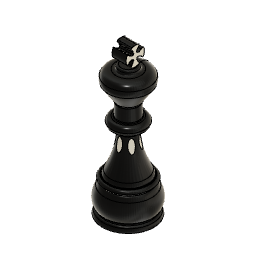
King (Autodesk Fusion 360 design; units mm, degrees)
Autodesk Fusion 360 part; units mm, degrees
(part 1 of 2)
sketch "King" plane through (0, 0, 0) normal (1, 0, 0) x (0, 1, 0)
  spline S0 degree 3 poles (88.295222, 49.849064) (89.98216, 50.061446) (91.649324, 49.850976) (93.310746, 49.908379) knots 0 0 0 0 1 1 1 1
  spline S1 degree 3 poles (93.310746, 49.908379) (93.855415, 49.926874) (93.710002, 49.535914) (93.695969, 49.290366) knots 0 0 0 0 1 1 1 1
  spline S2 degree 3 poles (93.695969, 49.290366) (93.638571, 48.352187) (93.519308, 47.4172) (93.457443, 46.479021) knots 0 0 0 0 1 1 1 1
  spline S3 degree 3 poles (93.457443, 46.479021) (93.421085, 45.919049) (93.415353, 45.480889) (94.299953, 45.59569) knots 0 0 0 0 1 1 1 1
  spline S4 degree 3 poles (94.299953, 45.59569) (94.931994, 45.677326) (95.640576, 45.650539) (96.29175, 45.57847) knots 0 0 0 0 1 1 1 1
  spline S5 degree 3 poles (96.29175, 45.57847) (97.320498, 45.464306) (97.41042, 45.937544) (97.282865, 46.743702) knots 0 0 0 0 1 1 1 1
  spline S6 degree 3 poles (97.282865, 46.743702) (97.158493, 47.528177) (97.128519, 48.328592) (96.995865, 49.11115) knots 0 0 0 0 1 1 1 1
  spline S7 degree 3 poles (96.995865, 49.11115) (96.893817, 49.711943) (97.141277, 49.926237) (97.686579, 49.925599) knots 0 0 0 0 1 1 1 1
  spline S8 degree 3 poles (97.686579, 49.925599) (99.190472, 49.923687) (100.69564, 49.921133) (102.198258, 49.912204) knots 0 0 0 0 1 1 1 1
  spline S9 degree 3 poles (102.198258, 49.912204) (102.707844, 49.909654) (102.999312, 49.79804) (102.885148, 49.134745) knots 0 0 0 0 1 1 1 1
  spline S10 degree 3 poles (102.885148, 49.134745) (102.473143, 46.743697) (101.897225, 44.366044) (100.371007, 42.473103) knots 0 0 0 0 1 1 1 1
  spline S11 degree 3 poles (100.371007, 42.473103) (99.617786, 41.540028) (98.842239, 40.438574) (97.084512, 40.530413) knots 0 0 0 0 1 1 1 1
  spline S12 degree 3 poles (97.084512, 40.530413) (92.929989, 40.747257) (88.756976, 40.584629) (84.591622, 40.565486) knots 0 0 0 0 1 1 1 1
  spline S13 degree 3 poles (84.591622, 40.565486) (83.961488, 40.562937) (83.402153, 40.683475) (82.942949, 41.155437) knots 0 0 0 0 1 1 1 1
  spline S14 degree 3 poles (82.942949, 41.155437) (80.750249, 43.416377) (79.704928, 46.184994) (79.359887, 49.260383) knots 0 0 0 0 1 1 1 1
  spline S15 degree 3 poles (79.359887, 49.260383) (79.326088, 49.555674) (79.183858, 49.961305) (79.775717, 49.951102) knots 0 0 0 0 1 1 1 1
  spline S16 degree 3 poles (79.775717, 49.951102) (81.317243, 49.924315) (82.860034, 49.928777) (84.402193, 49.924952) knots 0 0 0 0 1 1 1 1
  spline S17 degree 3 poles (84.402193, 49.924952) (84.984485, 49.92304) (85.252995, 49.714483) (85.154772, 49.063946) knots 0 0 0 0 1 1 1 1
  spline S18 degree 3 poles (85.154772, 49.063946) (85.015101, 48.136608) (84.967259, 47.195242) (84.870321, 46.26153) knots 0 0 0 0 1 1 1 1
  spline S19 degree 3 poles (84.870321, 46.26153) (84.830138, 45.887153) (84.860112, 45.517875) (85.334625, 45.564432) knots 0 0 0 0 1 1 1 1
  spline S20 degree 3 poles (85.334625, 45.564432) (86.334032, 45.663925) (87.34173, 45.403711) (88.341136, 45.668392) knots 0 0 0 0 1 1 1 1
  spline S21 degree 3 poles (88.341136, 45.668392) (88.594338, 45.735999) (88.788857, 45.702833) (88.752509, 46.051061) knots 0 0 0 0 1 1 1 1
  spline S22 degree 3 poles (88.752509, 46.051061) (88.619845, 47.303674) (88.682985, 48.578597) (88.295222, 49.849064) knots 0 0 0 0 1 1 1 1
  spline S23 degree 3 poles (32.804917, 55.77343) (30.85904, 55.684778) (28.973753, 57.437406) (28.855127, 59.445149) knots 0 0 0 0 1 1 1 1
  spline S24 degree 3 poles (28.855127, 59.445149) (28.719281, 61.741804) (30.431727, 63.767404) (32.57914, 63.848401) knots 0 0 0 0 1 1 1 1
  spline S25 degree 3 poles (32.57914, 63.848401) (34.856025, 63.933866) (36.967084, 62.39362) (36.930731, 59.527421) knots 0 0 0 0 1 1 1 1
  spline S26 degree 3 poles (36.930731, 59.527421) (36.909049, 57.853236) (35.523786, 55.816157) (32.804917, 55.77343) knots 0 0 0 0 1 1 1 1
  spline S27 degree 3 poles (-3.40457, 66.888069) (-2.853527, 66.263682) (-2.253372, 65.822973) (-1.529489, 65.53533) knots 0 0 0 0 1 1 1 1
  spline S28 degree 3 poles (-1.529489, 65.53533) (-1.252053, 65.424996) (-1.000768, 65.382901) (-0.766702, 65.520659) knots 0 0 0 0 1 1 1 1
  spline S29 degree 3 poles (-0.766702, 65.520659) (-0.442708, 65.713271) (-0.529445, 66.069153) (-0.5945, 66.342763) knots 0 0 0 0 1 1 1 1
  spline S30 degree 3 poles (-0.5945, 66.342763) (-0.736088, 66.937813) (-1.02564, 67.460157) (-1.505255, 67.870888) knots 0 0 0 0 1 1 1 1
  spline S31 degree 3 poles (-1.505255, 67.870888) (-1.91535, 68.222308) (-1.795447, 68.486346) (-1.331778, 68.68215) knots 0 0 0 0 1 1 1 1
  spline S32 degree 3 poles (-1.331778, 68.68215) (-0.632768, 68.976804) (0.116627, 69.05589) (0.833495, 68.955759) knots 0 0 0 0 1 1 1 1
  spline S33 degree 3 poles (0.833495, 68.955759) (2.154343, 68.770164) (2.208554, 68.532908) (1.445766, 67.461432) knots 0 0 0 0 1 1 1 1
  spline S34 degree 3 poles (1.445766, 67.461432) (1.069476, 66.932709) (0.436793, 66.287272) (1.044602, 65.686484) knots 0 0 0 0 1 1 1 1
  spline S35 degree 3 poles (1.044602, 65.686484) (1.70343, 65.034668) (2.367362, 65.740695) (2.894811, 66.132293) knots 0 0 0 0 1 1 1 1
  spline S36 degree 3 poles (2.894811, 66.132293) (3.795999, 66.80133) (4.067054, 66.782192) (4.250099, 65.699238) knots 0 0 0 0 1 1 1 1
  spline S37 degree 3 poles (4.250099, 65.699238) (4.392962, 64.851623) (4.480339, 63.975946) (4.074071, 63.130886) knots 0 0 0 0 1 1 1 1
  spline S38 degree 3 poles (4.074071, 63.130886) (3.839369, 62.642982) (3.686298, 62.435705) (3.265363, 62.970165) knots 0 0 0 0 1 1 1 1
  spline S39 degree 3 poles (3.265363, 62.970165) (2.882695, 63.454244) (2.348229, 63.767394) (1.75892, 63.931944) knots 0 0 0 0 1 1 1 1
  spline S40 degree 3 poles (1.75892, 63.931944) (1.06246, 64.12583) (0.724436, 63.78079) (0.87049, 63.076037) knots 0 0 0 0 1 1 1 1
  spline S41 degree 3 poles (0.87049, 63.076037) (1.013353, 62.387868) (1.479574, 61.888486) (1.897321, 61.366142) knots 0 0 0 0 1 1 1 1
  spline S42 degree 3 poles (1.897321, 61.366142) (2.223867, 60.957961) (2.184322, 60.770454) (1.632641, 60.628228) knots 0 0 0 0 1 1 1 1
  spline S43 degree 3 poles (1.632641, 60.628228) (0.702753, 60.387785) (-0.209914, 60.262143) (-1.138527, 60.583584) knots 0 0 0 0 1 1 1 1
  spline S44 degree 3 poles (-1.138527, 60.583584) (-1.749523, 60.795328) (-2.119436, 61.023018) (-1.449127, 61.670367) knots 0 0 0 0 1 1 1 1
  spline S45 degree 3 poles (-1.449127, 61.670367) (-1.077937, 62.028799) (-0.866832, 62.561352) (-0.617457, 63.03331) knots 0 0 0 0 1 1 1 1
  spline S46 degree 3 poles (-0.617457, 63.03331) (-0.483523, 63.287149) (-0.537734, 63.575424) (-0.729706, 63.787806) knots 0 0 0 0 1 1 1 1
  spline S47 degree 3 poles (-0.729706, 63.787806) (-0.92997, 64.009754) (-1.17743, 64.010392) (-1.462518, 63.889212) knots 0 0 0 0 1 1 1 1
  spline S48 degree 3 poles (-1.462518, 63.889212) (-2.044175, 63.641752) (-2.652621, 63.454244) (-3.078022, 62.939554) knots 0 0 0 0 1 1 1 1
  spline S49 degree 3 poles (-3.078022, 62.939554) (-3.416047, 62.530736) (-3.63417, 62.686352) (-3.768741, 63.111753) knots 0 0 0 0 1 1 1 1
  spline S50 degree 3 poles (-3.768741, 63.111753) (-4.167358, 64.373933) (-4.231775, 65.608679) (-3.40457, 66.888069) knots 0 0 0 0 1 1 1 1
  spline S51 degree 3 poles (134.32848, 40.360768) (132.205294, 41.878052) (130.602545, 43.799055) (129.497266, 46.158212) knots 0 0 0 0 1 1 1 1
  spline S52 degree 3 poles (129.497266, 46.158212) (129.186024, 46.822145) (128.865867, 47.537738) (128.279741, 47.989289) knots 0 0 0 0 1 1 1 1
  spline S53 degree 3 poles (128.279741, 47.989289) (127.659826, 48.466351) (127.314133, 48.86879) (127.629832, 49.724696) knots 0 0 0 0 1 1 1 1
  spline S54 degree 3 poles (127.629832, 49.724696) (127.886868, 50.42052) (127.423187, 51.113151) (126.876611, 51.455637) knots 0 0 0 0 1 1 1 1
  spline S55 degree 3 poles (126.876611, 51.455637) (126.403373, 51.752204) (126.004759, 51.185857) (125.676311, 50.811475) knots 0 0 0 0 1 1 1 1
  spline S56 degree 3 poles (125.676311, 50.811475) (125.337644, 50.426894) (124.966454, 50.359925) (124.427527, 50.451764) knots 0 0 0 0 1 1 1 1
  spline S57 degree 3 poles (124.427527, 50.451764) (121.666568, 50.923084) (119.036346, 50.471534) (116.559838, 49.154515) knots 0 0 0 0 1 1 1 1
  spline S58 degree 3 poles (116.559838, 49.154515) (114.237666, 47.919769) (112.702524, 46.003866) (111.62467, 43.63833) knots 0 0 0 0 1 1 1 1
  spline S59 degree 3 poles (111.62467, 43.63833) (110.243232, 40.608861) (109.600349, 37.40783) (109.385413, 34.123885) knots 0 0 0 0 1 1 1 1
  spline S60 degree 3 poles (109.385413, 34.123885) (109.150069, 30.51914) (109.299948, 26.913744) (110.003421, 23.361931) knots 0 0 0 0 1 1 1 1
  spline S61 degree 3 poles (110.003421, 23.361931) (110.380985, 21.456231) (110.852306, 19.571591) (111.717783, 17.794721) knots 0 0 0 0 1 1 1 1
  spline S62 degree 3 poles (111.717783, 17.794721) (112.014992, 17.181813) (112.370874, 16.874405) (112.900868, 16.769808) knots 0 0 0 0 1 1 1 1
  line L0 (112.900868, 16.769808) -> (128.298854, 16.769808)
  spline S63 degree 3 poles (128.298854, 16.769808) (128.712144, 16.855905) (128.881789, 17.128239) (128.935995, 17.633368) knots 0 0 0 0 1 1 1 1
  spline S64 degree 3 poles (128.935995, 17.633368) (129.147097, 19.555651) (129.375424, 21.475374) (129.624792, 23.391915) knots 0 0 0 0 1 1 1 1
  spline S65 degree 3 poles (129.624792, 23.391915) (129.697508, 23.948057) (129.53232, 24.320522) (129.118388, 24.708296) knots 0 0 0 0 1 1 1 1
  spline S66 degree 3 poles (129.118388, 24.708296) (127.229272, 26.471123) (125.479845, 28.356414) (124.242545, 30.660086) knots 0 0 0 0 1 1 1 1
  spline S67 degree 3 poles (124.242545, 30.660086) (122.998238, 32.979698) (122.026245, 35.380318) (121.938873, 38.058372) knots 0 0 0 0 1 1 1 1
  spline S68 degree 3 poles (121.938873, 38.058372) (121.92484, 38.469102) (122.016046, 39.016321) (122.367462, 39.04757) knots 0 0 0 0 1 1 1 1
  spline S69 degree 3 poles (122.367462, 39.04757) (122.838149, 39.08966) (122.728453, 38.509285) (122.7935, 38.170618) knots 0 0 0 0 1 1 1 1
  spline S70 degree 3 poles (122.7935, 38.170618) (123.213154, 35.969627) (124.448547, 35.266796) (126.661655, 35.799982) knots 0 0 0 0 1 1 1 1
  spline S71 degree 3 poles (126.661655, 35.799982) (128.582653, 36.262379) (130.517061, 36.572979) (132.13575, 34.857974) knots 0 0 0 0 1 1 1 1
  spline S72 degree 3 poles (132.13575, 34.857974) (132.348779, 34.632196) (133.05161, 34.012271) (133.616677, 34.937054) knots 0 0 0 0 1 1 1 1
  spline S73 degree 3 poles (133.616677, 34.937054) (134.08353, 35.698567) (134.68624, 36.385457) (135.069556, 37.214576) knots 0 0 0 0 1 1 1 1
  spline S74 degree 3 poles (135.069556, 37.214576) (135.723941, 38.62919) (135.575337, 39.469151) (134.32848, 40.360768) knots 0 0 0 0 1 1 1 1
  line L1 (102.334737, 3.260296) -> (79.669845, 3.260296)
  spline S75 degree 3 poles (79.669845, 3.260296) (78.967647, 3.011561) (78.601556, 2.40056) (78.233558, 1.257016) knots 0 0 0 0 1 1 1 1
  spline S76 degree 3 poles (78.233558, 1.257016) (77.972065, 0.443846) (78.199117, 0.343706) (78.894298, 0.345623) knots 0 0 0 0 1 1 1 1
  spline S77 degree 3 poles (78.894298, 0.345623) (82.659131, 0.359656) (86.423963, 0.359014) (90.188153, 0.356464) knots 0 0 0 0 1 1 1 1
  spline S78 degree 3 poles (90.188153, 0.356464) (94.570994, 0.353272) (98.951926, 0.354547) (103.332859, 0.325216) knots 0 0 0 0 1 1 1 1
  spline S79 degree 3 poles (103.332859, 0.325216) (104.040799, 0.320116) (104.111588, 0.614133) (103.980208, 1.194518) knots 0 0 0 0 1 1 1 1
  spline S80 degree 3 poles (103.980208, 1.194518) (103.707884, 2.394185) (103.22508, 3.025594) (102.334737, 3.260296) knots 0 0 0 0 1 1 1 1
  spline S81 degree 3 poles (38.99141, 16.190708) (39.060291, 16.192625) (39.129173, 16.195807) (39.19805, 16.199641) knots 0 0 0 0 1 1 1 1
  spline S82 degree 3 poles (39.19805, 16.199641) (39.19805, 16.196449) (39.19805, 16.193267) (39.19805, 16.190708) knots 0 0 0 0 1 1 1 1
  line L2 (39.19805, 16.190708) -> (41.8002, 16.190708)
  spline S83 degree 3 poles (41.8002, 16.190708) (42.145883, 17.004519) (41.415619, 17.417799) (41.11841, 17.961826) knots 0 0 0 0 1 1 1 1
  spline S84 degree 3 poles (41.11841, 17.961826) (38.833234, 22.135481) (37.535348, 26.59677) (36.994504, 31.315084) knots 0 0 0 0 1 1 1 1
  spline S85 degree 3 poles (36.994504, 31.315084) (36.870774, 32.396131) (36.972179, 33.513526) (36.581219, 34.669819) knots 0 0 0 0 1 1 1 1
  line L3 (36.581219, 34.669819) -> (28.943769, 34.669819)
  spline S86 degree 3 poles (28.943769, 34.669819) (28.773483, 34.470833) (28.714167, 34.199773) (28.696309, 33.859832) knots 0 0 0 0 1 1 1 1
  spline S87 degree 3 poles (28.696309, 33.859832) (28.545155, 30.988534) (28.07128, 28.161243) (27.40799, 25.367119) knots 0 0 0 0 1 1 1 1
  spline S88 degree 3 poles (27.40799, 25.367119) (26.631806, 22.092107) (24.830709, 19.246316) (23.532823, 16.190698) knots 0 0 0 0 1 1 1 1
  line L4 (23.532823, 16.190698) -> (38.99141, 16.190708)
  spline S89 degree 3 poles (42.254305, 15.822067) (42.187973, 15.826534) (42.091667, 15.824617) (41.998554, 15.828442) knots 0 0 0 0 1 1 1 1
  line L5 (41.998554, 15.828442) -> (23.18587, 15.828442)
  spline S90 degree 3 poles (23.18587, 15.828442) (23.118901, 15.813776) (23.04747, 15.808667) (22.976676, 15.808034) knots 0 0 0 0 1 1 1 1
  spline S91 degree 3 poles (22.976676, 15.808034) (22.224092, 15.801017) (21.936454, 15.235941) (21.968978, 14.682348) knots 0 0 0 0 1 1 1 1
  spline S92 degree 3 poles (21.968978, 14.682348) (22.010435, 13.994183) (22.542346, 13.769038) (23.270693, 13.771598) knots 0 0 0 0 1 1 1 1
  spline S93 degree 3 poles (23.270693, 13.771598) (29.545199, 13.792647) (35.820348, 13.775422) (42.09485, 13.759481) knots 0 0 0 0 1 1 1 1
  spline S94 degree 3 poles (42.09485, 13.759481) (42.725616, 13.758207) (43.304726, 13.900427) (43.386356, 14.585409) knots 0 0 0 0 1 1 1 1
  spline S95 degree 3 poles (43.386356, 14.585409) (43.475023, 15.334806) (43.04261, 15.77551) (42.254305, 15.822067) knots 0 0 0 0 1 1 1 1
  line L6 (83.250357, 37.423138) -> (98.576921, 37.423138)
  spline S96 degree 3 poles (98.576921, 37.423138) (98.641336, 37.430155) (98.704476, 37.435897) (98.768258, 37.446096) knots 0 0 0 0 1 1 1 1
  spline S97 degree 3 poles (98.768258, 37.446096) (99.605669, 37.575567) (100.289367, 38.34218) (100.172654, 39.018228) knots 0 0 0 0 1 1 1 1
  spline S98 degree 3 poles (100.172654, 39.018228) (100.026599, 39.866481) (99.518288, 40.270194) (98.631128, 40.26637) knots 0 0 0 0 1 1 1 1
  spline S99 degree 3 poles (98.631128, 40.26637) (93.665353, 40.240863) (88.699568, 40.230012) (83.734436, 40.230012) knots 0 0 0 0 1 1 1 1
  spline S100 degree 3 poles (83.734436, 40.230012) (83.081345, 40.230012) (82.538593, 40.070566) (82.266258, 39.448091) knots 0 0 0 0 1 1 1 1
  spline S101 degree 3 poles (82.266258, 39.448091) (81.891876, 38.592199) (82.384247, 37.714606) (83.250357, 37.423138) knots 0 0 0 0 1 1 1 1
  spline S102 degree 3 poles (99.326309, 26.046369) (98.959585, 29.268449) (98.668118, 32.494987) (98.36326, 35.721534) knots 0 0 0 0 1 1 1 1
  spline S103 degree 3 poles (98.36326, 35.721534) (98.275888, 36.648867) (98.229963, 36.960109) (97.7816, 37.060882) knots 0 0 0 0 1 1 1 1
  line L7 (97.7816, 37.060882) -> (84.371576, 37.060882)
  spline S104 degree 3 poles (84.371576, 37.060882) (84.171315, 36.991368) (84.023344, 36.822988) (83.992095, 36.410983) knots 0 0 0 0 1 1 1 1
  spline S105 degree 3 poles (83.992095, 36.410983) (83.836474, 34.269307) (83.612613, 32.132098) (83.405336, 29.994889) knots 0 0 0 0 1 1 1 1
  spline S106 degree 3 poles (83.405336, 29.994889) (83.071778, 26.559789) (82.728012, 23.125964) (82.382329, 19.613059) knots 0 0 0 0 1 1 1 1
  spline S107 degree 3 poles (82.382329, 19.613059) (84.224247, 19.613059) (86.098688, 19.615608) (87.974413, 19.613059) knots 0 0 0 0 1 1 1 1
  spline S108 degree 3 poles (87.974413, 19.613059) (91.568959, 19.609234) (95.162862, 19.625175) (98.756132, 19.58181) knots 0 0 0 0 1 1 1 1
  spline S109 degree 3 poles (98.756132, 19.58181) (99.610759, 19.570969) (99.849928, 19.854144) (99.786155, 20.684539) knots 0 0 0 0 1 1 1 1
  spline S110 degree 3 poles (99.786155, 20.684539) (99.650309, 22.474148) (99.528487, 24.276515) (99.326309, 26.046369) knots 0 0 0 0 1 1 1 1
  line L8 (-8.552116, 16.552331) -> (9.004772, 16.552331)
  spline S111 degree 3 poles (9.004772, 16.552331) (9.065362, 17.206697) (8.659094, 17.729042) (8.389314, 18.240545) knots 0 0 0 0 1 1 1 1
  spline S112 degree 3 poles (8.389314, 18.240545) (5.866881, 23.021999) (4.371922, 28.087914) (3.99499, 33.48292) knots 0 0 0 0 1 1 1 1
  spline S113 degree 3 poles (3.99499, 33.48292) (3.897409, 34.882858) (3.869348, 35.152633) (2.945839, 35.271263) knots 0 0 0 0 1 1 1 1
  line L9 (2.945839, 35.271263) -> (-3.592078, 35.271263)
  spline S114 degree 3 poles (-3.592078, 35.271263) (-3.815941, 35.209398) (-3.993882, 35.062711) (-3.995794, 34.707462) knots 0 0 0 0 1 1 1 1
  spline S115 degree 3 poles (-3.995794, 34.707462) (-3.997706, 34.169809) (-4.174372, 33.640448) (-4.184579, 33.127038) knots 0 0 0 0 1 1 1 1
  spline S116 degree 3 poles (-4.184579, 33.127038) (-4.240704, 30.330363) (-4.829378, 27.628077) (-5.501599, 24.936633) knots 0 0 0 0 1 1 1 1
  spline S117 degree 3 poles (-5.501599, 24.936633) (-6.141295, 22.376567) (-7.411758, 20.063329) (-8.387568, 17.635295) knots 0 0 0 0 1 1 1 1
  spline S118 degree 3 poles (-8.387568, 17.635295) (-8.550203, 17.230929) (-8.832739, 16.823391) (-8.552116, 16.552331) knots 0 0 0 0 1 1 1 1
  line L10 (-9.40228, 14.12238) -> (9.883636, 14.12238)
  spline S119 degree 3 poles (9.883636, 14.12238) (10.243985, 14.270985) (10.479324, 14.60136) (10.547568, 15.015915) knots 0 0 0 0 1 1 1 1
  spline S120 degree 3 poles (10.547568, 15.015915) (10.638132, 15.572057) (10.092831, 15.991722) (9.479917, 16.160101) knots 0 0 0 0 1 1 1 1
  spline S121 degree 3 poles (9.479917, 16.160101) (9.403382, 16.181784) (9.291772, 16.172217) (9.194829, 16.190075) knots 0 0 0 0 1 1 1 1
  line L11 (9.194829, 16.190075) -> (-8.991547, 16.190075)
  spline S122 degree 3 poles (-8.991547, 16.190075) (-9.00813, 16.188158) (-9.025351, 16.187525) (-9.042571, 16.18625) knots 0 0 0 0 1 1 1 1
  spline S123 degree 3 poles (-9.042571, 16.18625) (-9.768369, 16.141601) (-10.189943, 15.718754) (-10.169533, 15.029948) knots 0 0 0 0 1 1 1 1
  spline S124 degree 3 poles (-10.169533, 15.029948) (-10.152952, 14.501219) (-9.858295, 14.218044) (-9.40228, 14.12238) knots 0 0 0 0 1 1 1 1
  line L12 (-10.439952, 3.20609) -> (10.207632, 3.20609)
  spline S125 degree 3 poles (10.207632, 3.20609) (10.649616, 3.310045) (10.969145, 3.568988) (11.226171, 4.091333) knots 0 0 0 0 1 1 1 1
  spline S126 degree 3 poles (11.226171, 4.091333) (12.553398, 6.784052) (12.149679, 9.372174) (10.791841, 11.881848) knots 0 0 0 0 1 1 1 1
  spline S127 degree 3 poles (10.791841, 11.881848) (10.439784, 12.53239) (10.261205, 13.42209) (9.543699, 13.760124) knots 0 0 0 0 1 1 1 1
  line L13 (9.543699, 13.760124) -> (-4.066588, 13.760124)
  spline S128 degree 3 poles (-4.066588, 13.760124) (-4.775165, 13.738441) (-5.483104, 13.725683) (-6.185942, 13.760124) knots 0 0 0 0 1 1 1 1
  line L14 (-6.185942, 13.760124) -> (-8.636303, 13.760124)
  spline S129 degree 3 poles (-8.636303, 13.760124) (-9.638259, 13.515856) (-10.355128, 12.835973) (-10.977605, 11.66373) knots 0 0 0 0 1 1 1 1
  spline S130 degree 3 poles (-10.977605, 11.66373) (-12.372436, 9.0367) (-12.482135, 6.524476) (-11.168939, 3.890429) knots 0 0 0 0 1 1 1 1
  spline S131 degree 3 poles (-11.168939, 3.890429) (-10.982069, 3.513498) (-10.750552, 3.301753) (-10.439952, 3.20609) knots 0 0 0 0 1 1 1 1
  line L15 (10.477412, 2.845741) -> (-10.467377, 2.845741)
  spline S132 degree 3 poles (-10.467377, 2.845741) (-11.357084, 2.676729) (-11.952772, 1.88205) (-11.800343, 0.859043) knots 0 0 0 0 1 1 1 1
  spline S133 degree 3 poles (-11.800343, 0.859043) (-11.651101, -0.151204) (-10.762033, 0.484661) (-10.21354, 0.35264) knots 0 0 0 0 1 1 1 1
  spline S134 degree 3 poles (-10.21354, 0.35264) (-10.056006, 0.3131) (-9.880617, 0.344348) (-9.71288, 0.344348) knots 0 0 0 0 1 1 1 1
  spline S135 degree 3 poles (-9.71288, 0.344348) (-3.014247, 0.342431) (3.685665, 0.333507) (10.384935, 0.364123) knots 0 0 0 0 1 1 1 1
  spline S136 degree 3 poles (10.384935, 0.364123) (10.802045, 0.366041) (11.417508, 0.065639) (11.660501, 0.600742) knots 0 0 0 0 1 1 1 1
  spline S137 degree 3 poles (11.660501, 0.600742) (11.909236, 1.147319) (11.616494, 1.704104) (11.327576, 2.215607) knots 0 0 0 0 1 1 1 1
  spline S138 degree 3 poles (11.327576, 2.215607) (11.110732, 2.598913) (10.818628, 2.771117) (10.477412, 2.845741) knots 0 0 0 0 1 1 1 1
  line L16 (53.108731, 15.58864) -> (70.07121, 15.58864)
  spline S139 degree 3 poles (70.07121, 15.58864) (70.71091, 15.815693) (70.971761, 16.345686) (70.809123, 16.93628) knots 0 0 0 0 1 1 1 1
  spline S140 degree 3 poles (70.809123, 16.93628) (70.643303, 17.537705) (70.127333, 17.86553) (69.411745, 17.859156) knots 0 0 0 0 1 1 1 1
  spline S141 degree 3 poles (69.411745, 17.859156) (66.389292, 17.834924) (63.366198, 17.848947) (60.343113, 17.850864) knots 0 0 0 0 1 1 1 1
  spline S142 degree 3 poles (60.343113, 17.850864) (58.126181, 17.851506) (55.909249, 17.86298) (53.692317, 17.857881) knots 0 0 0 0 1 1 1 1
  spline S143 degree 3 poles (53.692317, 17.857881) (52.865115, 17.855331) (52.437159, 17.36551) (52.435884, 16.588689) knots 0 0 0 0 1 1 1 1
  spline S144 degree 3 poles (52.435884, 16.588689) (52.433957, 16.030629) (52.692258, 15.718745) (53.108731, 15.58864) knots 0 0 0 0 1 1 1 1
  line L17 (81.065948, 16.795325) -> (82.356822, 16.795325)
  spline S145 degree 3 poles (82.356822, 16.795325) (82.371488, 16.795325) (82.385521, 16.795325) (82.400187, 16.795325) knots 0 0 0 0 1 1 1 1
  line L18 (82.400187, 16.795325) -> (100.817443, 16.795325)
  spline S146 degree 3 poles (100.817443, 16.795325) (101.737127, 16.898647) (102.239064, 17.32596) (102.210997, 17.986068) knots 0 0 0 0 1 1 1 1
  spline S147 degree 3 poles (102.210997, 17.986068) (102.176557, 18.798605) (101.535582, 19.243134) (100.388855, 19.246968) knots 0 0 0 0 1 1 1 1
  spline S148 degree 3 poles (100.388855, 19.246968) (98.885604, 19.253342) (97.381069, 19.254617) (95.877818, 19.258452) knots 0 0 0 0 1 1 1 1
  spline S149 degree 3 poles (95.877818, 19.258452) (92.237358, 19.264826) (88.59753, 19.275034) (84.956418, 19.276309) knots 0 0 0 0 1 1 1 1
  spline S150 degree 3 poles (84.956418, 19.276309) (83.857514, 19.278227) (82.759894, 19.258452) (81.660999, 19.245693) knots 0 0 0 0 1 1 1 1
  spline S151 degree 3 poles (81.660999, 19.245693) (80.775756, 19.234852) (80.338876, 18.661484) (80.333135, 17.899338) knots 0 0 0 0 1 1 1 1
  spline S152 degree 3 poles (80.333135, 17.899338) (80.328668, 17.339994) (80.574853, 16.940737) (81.065948, 16.795325) knots 0 0 0 0 1 1 1 1
  spline S153 degree 3 poles (103.85967, 11.717303) (103.245487, 13.225021) (102.306671, 14.536945) (101.540691, 15.951539) knots 0 0 0 0 1 1 1 1
  spline S154 degree 3 poles (101.540691, 15.951539) (101.307264, 16.382677) (100.916299, 16.412661) (100.501744, 16.412018) knots 0 0 0 0 1 1 1 1
  spline S155 degree 3 poles (100.501744, 16.412018) (99.327583, 16.412018) (98.15279, 16.411376) (96.97863, 16.411376) knots 0 0 0 0 1 1 1 1
  spline S156 degree 3 poles (96.97863, 16.411376) (95.85996, 16.410734) (94.741923, 16.411376) (93.623895, 16.411376) knots 0 0 0 0 1 1 1 1
  spline S157 degree 3 poles (93.623895, 16.411376) (93.623895, 16.419025) (93.623895, 16.425409) (93.623895, 16.433058) knots 0 0 0 0 1 1 1 1
  line L19 (93.623895, 16.433058) -> (81.79557, 16.433058)
  spline S158 degree 3 poles (81.79557, 16.433058) (81.647608, 16.402442) (81.515587, 16.333561) (81.410989, 16.180499) knots 0 0 0 0 1 1 1 1
  spline S159 degree 3 poles (81.410989, 16.180499) (80.39245, 14.690639) (79.320979, 13.221829) (78.46316, 11.64012) knots 0 0 0 0 1 1 1 1
  spline S160 degree 3 poles (78.46316, 11.64012) (77.414005, 9.704447) (77.792212, 7.646961) (78.498234, 5.694072) knots 0 0 0 0 1 1 1 1
  spline S161 degree 3 poles (78.498234, 5.694072) (78.986137, 4.343882) (79.295462, 3.857896) (80.14244, 3.713116) knots 0 0 0 0 1 1 1 1
  line L20 (80.14244, 3.713116) -> (102.388311, 3.713116)
  spline S162 degree 3 poles (102.388311, 3.713116) (102.60388, 3.795389) (102.799683, 3.950368) (102.956579, 4.232268) knots 0 0 0 0 1 1 1 1
  spline S163 degree 3 poles (102.956579, 4.232268) (104.27551, 6.601639) (104.953466, 9.032875) (103.85967, 11.717303) knots 0 0 0 0 1 1 1 1
  spline S164 degree 3 poles (43.284328, 3.087459) (44.286285, 3.466941) (44.479529, 4.558186) (44.741664, 5.493178) knots 0 0 0 0 1 1 1 1
  spline S165 degree 3 poles (44.741664, 5.493178) (45.498078, 8.193547) (44.464863, 10.548884) (43.138916, 12.827682) knots 0 0 0 0 1 1 1 1
  spline S166 degree 3 poles (43.138916, 12.827682) (42.81109, 13.392116) (42.431619, 13.556029) (41.767686, 13.552204) knots 0 0 0 0 1 1 1 1
  spline S167 degree 3 poles (41.767686, 13.552204) (35.650071, 13.517763) (29.53246, 13.520955) (23.414845, 13.560495) knots 0 0 0 0 1 1 1 1
  spline S168 degree 3 poles (23.414845, 13.560495) (22.808953, 13.56432) (22.415438, 13.35385) (22.169253, 12.913146) knots 0 0 0 0 1 1 1 1
  spline S169 degree 3 poles (22.169253, 12.913146) (21.660942, 12.001121) (20.97341, 11.20835) (20.5799, 10.212777) knots 0 0 0 0 1 1 1 1
  spline S170 degree 3 poles (20.5799, 10.212777) (19.561361, 7.638046) (20.012911, 5.3095) (21.465781, 3.087469) knots 0 0 0 0 1 1 1 1
  line L21 (21.465781, 3.087469) -> (43.284328, 3.087459)
  line L22 (43.536888, 2.72456) -> (21.365003, 2.72456)
  spline S171 degree 3 poles (21.365003, 2.72456) (21.200453, 2.590622) (21.028254, 2.450318) (20.863066, 2.298522) knots 0 0 0 0 1 1 1 1
  spline S172 degree 3 poles (20.863066, 2.298522) (20.363047, 1.841867) (20.229108, 1.183044) (20.405774, 0.632633) knots 0 0 0 0 1 1 1 1
  spline S173 degree 3 poles (20.405774, 0.632633) (20.574786, 0.10264) (21.229152, 0.37369) (21.66157, 0.369233) knots 0 0 0 0 1 1 1 1
  spline S174 degree 3 poles (21.66157, 0.369233) (24.543709, 0.341166) (27.425853, 0.338616) (30.308629, 0.342441) knots 0 0 0 0 1 1 1 1
  spline S175 degree 3 poles (30.308629, 0.342441) (34.847728, 0.348815) (39.386194, 0.383256) (43.924661, 0.358382) knots 0 0 0 0 1 1 1 1
  spline S176 degree 3 poles (43.924661, 0.358382) (44.755688, 0.353282) (44.735923, 0.638365) (44.6326, 1.315056) knots 0 0 0 0 1 1 1 1
  spline S177 degree 3 poles (44.6326, 1.315056) (44.508238, 2.135252) (44.097497, 2.51919) (43.536888, 2.72456) knots 0 0 0 0 1 1 1 1
  line L23 (111.847265, 14.317541) -> (129.331437, 14.317541)
  spline S178 degree 3 poles (129.331437, 14.317541) (129.754283, 14.583502) (130.096141, 14.940016) (129.871629, 15.587366) knots 0 0 0 0 1 1 1 1
  spline S179 degree 3 poles (129.871629, 15.587366) (129.594837, 16.383952) (128.907948, 16.426052) (128.214674, 16.424777) knots 0 0 0 0 1 1 1 1
  spline S180 degree 3 poles (128.214674, 16.424777) (128.079461, 16.424777) (127.946174, 16.419677) (127.81096, 16.420952) knots 0 0 0 0 1 1 1 1
  spline S181 degree 3 poles (127.81096, 16.420952) (124.461316, 16.424777) (121.110415, 16.434985) (117.760138, 16.433068) knots 0 0 0 0 1 1 1 1
  spline S182 degree 3 poles (117.760138, 16.433068) (116.014526, 16.432426) (114.268915, 16.406919) (112.523303, 16.402452) knots 0 0 0 0 1 1 1 1
  spline S183 degree 3 poles (112.523303, 16.402452) (111.734366, 16.40181) (111.160366, 16.050395) (111.155899, 15.252533) knots 0 0 0 0 1 1 1 1
  spline S184 degree 3 poles (111.155899, 15.252533) (111.153359, 14.716788) (111.443551, 14.443821) (111.847265, 14.317541) knots 0 0 0 0 1 1 1 1
  spline S185 degree 3 poles (129.421378, 2.880182) (128.356914, 2.879539) (127.29245, 2.880182) (126.228006, 2.880182) knots 0 0 0 0 1 1 1 1
  spline S186 degree 3 poles (126.228006, 2.880182) (126.228006, 2.882731) (126.228006, 2.884006) (126.228006, 2.886556) knots 0 0 0 0 1 1 1 1
  line L24 (126.228006, 2.886556) -> (114.092906, 2.886556)
  spline S187 degree 3 poles (114.092906, 2.886556) (113.658576, 2.85594) (113.224888, 2.830433) (112.795657, 2.886556) knots 0 0 0 0 1 1 1 1
  line L25 (112.795657, 2.886556) -> (111.393812, 2.886556)
  spline S188 degree 3 poles (111.393812, 2.886556) (111.339596, 2.876347) (111.279016, 2.876347) (111.213316, 2.886556) knots 0 0 0 0 1 1 1 1
  line L26 (111.212041, 2.886556) -> (110.808328, 2.886556)
  spline S189 degree 3 poles (110.808328, 2.886556) (110.27195, 2.795992) (109.991966, 2.330413) (109.768106, 1.866742) knots 0 0 0 0 1 1 1 1
  spline S190 degree 3 poles (109.768106, 1.866742) (109.25852, 0.816953) (109.603561, 0.337974) (110.757946, 0.362216) knots 0 0 0 0 1 1 1 1
  spline S191 degree 3 poles (110.757946, 0.362216) (111.293681, 0.374332) (111.830059, 0.361574) (112.366437, 0.361574) knots 0 0 0 0 1 1 1 1
  spline S192 degree 3 poles (112.366437, 0.361574) (118.336727, 0.358382) (124.308293, 0.355832) (130.279216, 0.358382) knots 0 0 0 0 1 1 1 1
  spline S193 degree 3 poles (130.279216, 0.358382) (130.594273, 0.359024) (130.960364, 0.260159) (131.076445, 0.74488) knots 0 0 0 0 1 1 1 1
  spline S194 degree 3 poles (131.076445, 0.74488) (131.314309, 1.732803) (130.436093, 2.882089) (129.421378, 2.880182) knots 0 0 0 0 1 1 1 1
  line L27 (129.176467, 13.955275) -> (112.039244, 13.955275)
  spline S195 degree 3 poles (112.039244, 13.955275) (111.61703, 13.757564) (111.305798, 13.343642) (111.000297, 12.852546) knots 0 0 0 0 1 1 1 1
  spline S196 degree 3 poles (111.000297, 12.852546) (110.668647, 12.319361) (110.412896, 11.761933) (110.132279, 11.211532) knots 0 0 0 0 1 1 1 1
  spline S197 degree 3 poles (110.132279, 11.211532) (108.933244, 8.875337) (109.059524, 6.542324) (110.109322, 4.186354) knots 0 0 0 0 1 1 1 1
  spline S198 degree 3 poles (110.109322, 4.186354) (110.317242, 3.717583) (110.564702, 3.378917) (110.930783, 3.248812) knots 0 0 0 0 1 1 1 1
  line L28 (110.930783, 3.248812) -> (111.708236, 3.248812)
  spline S199 degree 3 poles (111.708236, 3.248812) (111.711428, 3.248812) (111.714611, 3.250087) (111.715886, 3.250729) knots 0 0 0 0 1 1 1 1
  spline S200 degree 3 poles (111.715886, 3.250729) (111.716528, 3.251372) (111.716528, 3.253279) (111.716528, 3.254554) knots 0 0 0 0 1 1 1 1
  spline S201 degree 3 poles (111.716528, 3.254554) (111.71972, 3.253279) (111.721627, 3.251362) (111.723545, 3.250729) knots 0 0 0 0 1 1 1 1
  spline S202 degree 3 poles (111.723545, 3.250729) (112.988902, 3.250729) (114.254269, 3.250729) (115.519626, 3.250729) knots 0 0 0 0 1 1 1 1
  spline S203 degree 2 poles (115.519626, 3.250729) (115.519626, 3.250087) (115.519626, 3.248812) knots 0 0 0 1 1 1
  line L29 (115.519626, 3.248812) -> (129.779177, 3.248812)
  spline S204 degree 3 poles (129.779177, 3.248812) (130.072552, 3.336827) (130.285581, 3.533905) (130.443099, 3.850879) knots 0 0 0 0 1 1 1 1
  spline S205 degree 3 poles (130.443099, 3.850879) (130.909311, 4.783322) (131.296461, 5.72787) (131.377449, 6.80445) knots 0 0 0 0 1 1 1 1
  spline S206 degree 3 poles (131.377449, 6.80445) (131.576445, 9.476772) (130.58277, 11.742168) (129.176467, 13.955275) knots 0 0 0 0 1 1 1 1
  line L30 (111.715244, 3.250731) -> (111.715244, 3.248818)
  line L31 (111.715244, 3.248818) -> (111.726086, 3.248818)
  line L32 (111.726086, 3.248818) -> (111.722259, 3.250731)
  line L33 (111.722259, 3.250731) -> (111.715886, 3.250729)
  line L34 (111.715886, 3.250729) -> (111.715244, 3.250731)
  spline S207 degree 3 poles (66.523221, 40.033585) (66.037868, 40.46919) (66.231122, 40.634378) (66.490698, 41.051482) knots 0 0 0 0 1 1 1 1
  spline S208 degree 3 poles (66.490698, 41.051482) (67.871493, 43.267782) (68.387464, 45.548491) (67.021334, 48.0199) knots 0 0 0 0 1 1 1 1
  spline S209 degree 3 poles (67.021334, 48.0199) (65.838882, 50.159021) (64.508467, 52.192913) (63.047949, 54.145807) knots 0 0 0 0 1 1 1 1
  spline S210 degree 3 poles (63.047949, 54.145807) (62.83238, 54.432807) (62.715666, 54.661772) (62.787098, 54.92964) knots 0 0 0 0 1 1 1 1
  spline S211 degree 3 poles (62.787098, 54.92964) (63.348982, 55.297) (63.721447, 55.930959) (63.721447, 56.652931) knots 0 0 0 0 1 1 1 1
  spline S212 degree 3 poles (63.721447, 56.652931) (63.721447, 57.790096) (62.800489, 58.711692) (61.662686, 58.711692) knots 0 0 0 0 1 1 1 1
  spline S213 degree 3 poles (61.662686, 58.711692) (60.524884, 58.711692) (59.603925, 57.790096) (59.603925, 56.652931) knots 0 0 0 0 1 1 1 1
  spline S214 degree 3 poles (59.603925, 56.652931) (59.603925, 55.935425) (59.971923, 55.304022) (60.528076, 54.936019) knots 0 0 0 0 1 1 1 1
  spline S215 degree 3 poles (60.528076, 54.936019) (60.5791, 54.46916) (60.252549, 54.092871) (59.943866, 53.665557) knots 0 0 0 0 1 1 1 1
  spline S216 degree 3 poles (59.943866, 53.665557) (59.70789, 53.339012) (59.485304, 53.00035) (59.224443, 52.694212) knots 0 0 0 0 1 1 1 1
  spline S217 degree 3 poles (59.224443, 52.694212) (58.682966, 52.060896) (58.591127, 51.438417) (59.016524, 50.671167) knots 0 0 0 0 1 1 1 1
  spline S218 degree 3 poles (59.016524, 50.671167) (59.485295, 49.822277) (59.838627, 48.90706) (60.225125, 48.013526) knots 0 0 0 0 1 1 1 1
  spline S219 degree 3 poles (60.225125, 48.013526) (60.309947, 47.817727) (60.477685, 47.537101) (60.156243, 47.408271) knots 0 0 0 0 1 1 1 1
  spline S220 degree 3 poles (60.156243, 47.408271) (59.887733, 47.301124) (59.727013, 47.529452) (59.612849, 47.741196) knots 0 0 0 0 1 1 1 1
  spline S221 degree 3 poles (59.612849, 47.741196) (59.519093, 47.918499) (59.471261, 48.123227) (59.366664, 48.294152) knots 0 0 0 0 1 1 1 1
  spline S222 degree 3 poles (59.366664, 48.294152) (58.88641, 49.07416) (58.742272, 50.041675) (58.070048, 50.758544) knots 0 0 0 0 1 1 1 1
  spline S223 degree 3 poles (58.070048, 50.758544) (57.714799, 50.299339) (57.352543, 49.937716) (57.119116, 49.506578) knots 0 0 0 0 1 1 1 1
  spline S224 degree 3 poles (57.119116, 49.506578) (56.372269, 48.124502) (55.310364, 46.89996) (55.443661, 45.122458) knots 0 0 0 0 1 1 1 1
  spline S225 degree 3 poles (55.443661, 45.122458) (55.564841, 43.524176) (56.108868, 42.147205) (56.977528, 40.856963) knots 0 0 0 0 1 1 1 1
  spline S226 degree 3 poles (56.977528, 40.856963) (57.115291, 40.652868) (57.26772, 40.53233) (57.0834, 40.257446) knots 0 0 0 0 1 1 1 1
  spline S227 degree 3 poles (57.0834, 40.257446) (56.27788, 39.057136) (56.295738, 38.506093) (57.470531, 38.131078) knots 0 0 0 0 1 1 1 1
  line L35 (57.470531, 38.131078) -> (66.0755, 38.131078)
  spline S228 degree 3 poles (66.0755, 38.131078) (66.088259, 38.135545) (66.099733, 38.139369) (66.111216, 38.145111) knots 0 0 0 0 1 1 1 1
  spline S229 degree 3 poles (66.111216, 38.145111) (66.99136, 38.585815) (67.222237, 39.406644) (66.523221, 40.033585) knots 0 0 0 0 1 1 1 1
  line L36 (52.547488, 3.449083) -> (70.244047, 3.449083)
  spline S230 degree 3 poles (70.244047, 3.449083) (70.688585, 3.543471) (70.985785, 3.803048) (71.233887, 4.306259) knots 0 0 0 0 1 1 1 1
  spline S231 degree 3 poles (71.233887, 4.306259) (72.628716, 7.137375) (72.65359, 9.927675) (71.257487, 12.774741) knots 0 0 0 0 1 1 1 1
  spline S232 degree 3 poles (71.257487, 12.774741) (70.85823, 13.589827) (70.264454, 14.325191) (70.044428, 15.226374) knots 0 0 0 0 1 1 1 1
  line L37 (70.044428, 15.226374) -> (55.151561, 15.226374)
  spline S233 degree 3 poles (55.151561, 15.226374) (55.085871, 15.219358) (55.022731, 15.219358) (54.959591, 15.226374) knots 0 0 0 0 1 1 1 1
  line L38 (54.959591, 15.226374) -> (53.761199, 15.226374)
  spline S234 degree 3 poles (53.761199, 15.226374) (52.978003, 14.997414) (52.537289, 14.262683) (52.046836, 13.40359) knots 0 0 0 0 1 1 1 1
  spline S235 degree 3 poles (52.046836, 13.40359) (50.368189, 10.462768) (50.209386, 7.537264) (51.557015, 4.467612) knots 0 0 0 0 1 1 1 1
  spline S236 degree 3 poles (51.557015, 4.467612) (51.791717, 3.932519) (52.072333, 3.571538) (52.547488, 3.449083) knots 0 0 0 0 1 1 1 1
  line L39 (70.46345, 3.087459) -> (57.756266, 3.087459)
  spline S237 degree 3 poles (57.756266, 3.087459) (57.407401, 3.057485) (57.048327, 3.037078) (56.68862, 3.087459) knots 0 0 0 0 1 1 1 1
  line L40 (56.68862, 3.087459) -> (52.699927, 3.087459)
  spline S238 degree 3 poles (52.699927, 3.087459) (51.659063, 2.941404) (51.2477, 2.478375) (51.118861, 1.30549) knots 0 0 0 0 1 1 1 1
  spline S239 degree 3 poles (51.118861, 1.30549) (51.046787, 0.63964) (51.203683, 0.353282) (51.978597, 0.359656) knots 0 0 0 0 1 1 1 1
  spline S240 degree 3 poles (51.978597, 0.359656) (55.927107, 0.394097) (59.877535, 0.357739) (63.827329, 0.35519) knots 0 0 0 0 1 1 1 1
  spline S241 degree 3 poles (63.827329, 0.35519) (66.206899, 0.35264) (68.588376, 0.363481) (70.967314, 0.37369) knots 0 0 0 0 1 1 1 1
  spline S242 degree 3 poles (70.967314, 0.37369) (71.283013, 0.374332) (71.631888, 0.265268) (71.733293, 0.781238) knots 0 0 0 0 1 1 1 1
  spline S243 degree 3 poles (71.733293, 0.781238) (71.920144, 1.732803) (71.331468, 2.790892) (70.46345, 3.087459) knots 0 0 0 0 1 1 1 1
  spline S244 degree 3 poles (39.981887, 54.968547) (38.736295, 54.291862) (37.509204, 54.204485) (36.356731, 54.949415) knots 0 0 0 0 1 1 1 1
  spline S245 degree 3 poles (36.356731, 54.949415) (35.671753, 55.392036) (35.256556, 55.353133) (34.574129, 54.959618) knots 0 0 0 0 1 1 1 1
  spline S246 degree 3 poles (34.574129, 54.959618) (33.376373, 54.268262) (32.097615, 53.958299) (30.83927, 55.009367) knots 0 0 0 0 1 1 1 1
  spline S247 degree 3 poles (30.83927, 55.009367) (30.543978, 55.25619) (30.121764, 55.58911) (29.576458, 55.222387) knots 0 0 0 0 1 1 1 1
  spline S248 degree 3 poles (29.576458, 55.222387) (28.188003, 54.289949) (26.752992, 54.269537) (25.259945, 55.066128) knots 0 0 0 0 1 1 1 1
  spline S249 degree 3 poles (25.259945, 55.066128) (24.206327, 55.628013) (23.185875, 55.253635) (22.507272, 54.182797) knots 0 0 0 0 1 1 1 1
  spline S250 degree 3 poles (22.507272, 54.182797) (21.993857, 53.37409) (22.189018, 52.263707) (23.060865, 51.578092) knots 0 0 0 0 1 1 1 1
  spline S251 degree 3 poles (23.060865, 51.578092) (26.525302, 48.852844) (27.711578, 45.039543) (28.142721, 40.895861) knots 0 0 0 0 1 1 1 1
  spline S252 degree 3 poles (28.142721, 40.895861) (28.262627, 39.741476) (28.273468, 39.295662) (27.821917, 39.108792) knots 0 0 0 0 1 1 1 1
  line L41 (27.821917, 39.108792) -> (25.996583, 39.108792)
  spline S253 degree 3 poles (25.996583, 39.108792) (24.870259, 39.108792) (23.956955, 38.195483) (23.956955, 37.069796) knots 0 0 0 0 1 1 1 1
  spline S254 degree 3 poles (23.956955, 37.069796) (23.956955, 36.005333) (24.772678, 35.132216) (25.812905, 35.039092) knots 0 0 0 0 1 1 1 1
  spline S255 degree 3 poles (25.812905, 35.039092) (25.825021, 35.037175) (25.837142, 35.03335) (25.849258, 35.030158) knots 0 0 0 0 1 1 1 1
  line L42 (25.849258, 35.030158) -> (25.996588, 35.030158)
  line L43 (25.996588, 35.030158) -> (38.955699, 35.030158)
  line L44 (38.955699, 35.030158) -> (39.010547, 35.030158)
  spline S256 degree 3 poles (39.010547, 35.030158) (39.020751, 35.031433) (39.02968, 35.03335) (39.039246, 35.034625) knots 0 0 0 0 1 1 1 1
  spline S257 degree 3 poles (39.039246, 35.034625) (39.41809, 35.049933) (39.770148, 35.167279) (40.068627, 35.36245) knots 0 0 0 0 1 1 1 1
  spline S258 degree 3 poles (40.068627, 35.36245) (40.425784, 35.569095) (40.682173, 35.856728) (40.800166, 36.204961) knots 0 0 0 0 1 1 1 1
  spline S259 degree 3 poles (40.800166, 36.204961) (40.923891, 36.467729) (40.99469, 36.760471) (40.99469, 37.069796) knots 0 0 0 0 1 1 1 1
  spline S260 degree 3 poles (40.99469, 37.069796) (40.99469, 38.196125) (40.082023, 39.108792) (38.955699, 39.108792) knots 0 0 0 0 1 1 1 1
  line L45 (38.955699, 39.108792) -> (37.442877, 39.108792)
  spline S261 degree 3 poles (37.442877, 39.108792) (37.265573, 39.27398) (37.277052, 39.609454) (37.302564, 40.291244) knots 0 0 0 0 1 1 1 1
  spline S262 degree 3 poles (37.302564, 40.291244) (37.305113, 40.358209) (37.295547, 40.425816) (37.299377, 40.492147) knots 0 0 0 0 1 1 1 1
  spline S263 degree 3 poles (37.299377, 40.492147) (37.574261, 44.792715) (38.847277, 48.63727) (42.27408, 51.525151) knots 0 0 0 0 1 1 1 1
  spline S264 degree 3 poles (42.27408, 51.525151) (42.718619, 51.899529) (43.151674, 52.350442) (43.171439, 53.029044) knots 0 0 0 0 1 1 1 1
  spline S265 degree 3 poles (43.171439, 53.029044) (43.221821, 54.791881) (41.580174, 55.837207) (39.981887, 54.968547) knots 0 0 0 0 1 1 1 1
  line L46 (-33.913553, 13.043251) -> (-17.134123, 13.043251)
  spline S266 degree 3 poles (-17.134123, 13.043251) (-16.736784, 13.209713) (-16.448506, 13.506922) (-16.552466, 14.01714) knots 0 0 0 0 1 1 1 1
  spline S267 degree 3 poles (-16.552466, 14.01714) (-16.657063, 14.531193) (-16.915365, 14.759521) (-17.245737, 14.864118) knots 0 0 0 0 1 1 1 1
  line L47 (-17.245737, 14.864118) -> (-33.685227, 14.864118)
  spline S268 degree 3 poles (-33.685227, 14.864118) (-34.084479, 14.691914) (-34.289845, 14.320091) (-34.301325, 13.772872) knots 0 0 0 0 1 1 1 1
  spline S269 degree 3 poles (-34.301325, 13.772872) (-34.310254, 13.350026) (-34.152721, 13.143381) (-33.913553, 13.043251) knots 0 0 0 0 1 1 1 1
  line L48 (-34.504778, 2.951613) -> (-16.560118, 2.951613)
  spline S270 degree 3 poles (-16.560118, 2.951613) (-16.072851, 3.232239) (-15.831771, 3.803057) (-15.595789, 4.394274) knots 0 0 0 0 1 1 1 1
  spline S271 degree 3 poles (-15.595789, 4.394274) (-14.823435, 6.321656) (-15.077272, 8.213322) (-15.834958, 10.058421) knots 0 0 0 0 1 1 1 1
  spline S272 degree 3 poles (-15.834958, 10.058421) (-16.221453, 10.999788) (-16.617518, 11.960929) (-17.39051, 12.680984) knots 0 0 0 0 1 1 1 1
  line L49 (-17.39051, 12.680984) -> (-33.695431, 12.680984)
  spline S273 degree 3 poles (-33.695431, 12.680984) (-33.752194, 12.648461) (-33.80513, 12.605728) (-33.852326, 12.543221) knots 0 0 0 0 1 1 1 1
  spline S274 degree 3 poles (-33.852326, 12.543221) (-35.633016, 10.173218) (-36.777836, 7.65206) (-35.688503, 4.616859) knots 0 0 0 0 1 1 1 1
  spline S275 degree 3 poles (-35.688503, 4.616859) (-35.308384, 3.557505) (-35.08516, 3.123175) (-34.504778, 2.951613) knots 0 0 0 0 1 1 1 1
  line L50 (-16.512283, 2.589989) -> (-34.845353, 2.589989)
  spline S276 degree 3 poles (-34.845353, 2.589989) (-35.508648, 2.37442) (-35.891955, 1.712395) (-35.813508, 0.882011) knots 0 0 0 0 1 1 1 1
  spline S277 degree 3 poles (-35.813508, 0.882011) (-35.725494, -0.051707) (-34.96717, 0.377524) (-34.556438, 0.372425) knots 0 0 0 0 1 1 1 1
  spline S278 degree 3 poles (-34.556438, 0.372425) (-30.868777, 0.329692) (-27.180479, 0.352017) (-23.492817, 0.355842) knots 0 0 0 0 1 1 1 1
  spline S279 degree 3 poles (-23.492817, 0.355842) (-21.020132, 0.357116) (-18.546172, 0.376891) (-16.073489, 0.355842) knots 0 0 0 0 1 1 1 1
  spline S280 degree 3 poles (-16.073489, 0.355842) (-15.457391, 0.349467) (-15.326644, 0.559937) (-15.452289, 1.133295) knots 0 0 0 0 1 1 1 1
  spline S281 degree 3 poles (-15.452289, 1.133295) (-15.631505, 1.955398) (-15.88088, 2.366129) (-16.512283, 2.589989) knots 0 0 0 0 1 1 1 1
  spline S282 degree 3 poles (-22.307179, 28.109597) (-22.458333, 28.755671) (-22.483207, 29.045863) (-22.252329, 29.174693) knots 0 0 0 0 1 1 1 1
  line L51 (-22.252329, 29.174693) -> (-19.889982, 29.174693)
  spline S283 degree 3 poles (-19.889982, 29.174693) (-18.545535, 29.174693) (-17.455564, 30.264664) (-17.455564, 31.609744) knots 0 0 0 0 1 1 1 1
  spline S284 degree 3 poles (-17.455564, 31.609744) (-17.455564, 32.954191) (-18.545535, 34.044794) (-19.889982, 34.044794) knots 0 0 0 0 1 1 1 1
  line L52 (-19.889982, 34.044794) -> (-22.34162, 34.044794)
  spline S285 degree 3 poles (-22.34162, 34.044794) (-22.36458, 34.052444) (-22.386902, 34.058828) (-22.409225, 34.067119) knots 0 0 0 0 1 1 1 1
  spline S286 degree 3 poles (-22.409225, 34.067119) (-18.395658, 36.93395) (-18.824249, 41.536836) (-21.148967, 44.015257) knots 0 0 0 0 1 1 1 1
  spline S287 degree 3 poles (-21.148967, 44.015257) (-23.393324, 46.40758) (-27.617998, 46.672898) (-30.185075, 43.975074) knots 0 0 0 0 1 1 1 1
  spline S288 degree 3 poles (-30.185075, 43.975074) (-32.194729, 41.863377) (-33.136735, 37.407821) (-28.889738, 34.044794) knots 0 0 0 0 1 1 1 1
  line L53 (-28.889738, 34.044794) -> (-31.481688, 34.044794)
  spline S289 degree 3 poles (-31.481688, 34.044794) (-32.826134, 34.044794) (-33.916743, 32.954181) (-33.916743, 31.609744) knots 0 0 0 0 1 1 1 1
  spline S290 degree 3 poles (-33.916743, 31.609744) (-33.916743, 30.264664) (-32.826134, 29.174693) (-31.481688, 29.174693) knots 0 0 0 0 1 1 1 1
  line L54 (-31.481688, 29.174693) -> (-29.188858, 29.174693)
  spline S291 degree 3 poles (-29.188858, 29.174693) (-28.730293, 29.022896) (-28.801086, 28.623007) (-29.070869, 27.560461) knots 0 0 0 0 1 1 1 1
  spline S292 degree 3 poles (-29.070869, 27.560461) (-30.067086, 23.629808) (-31.098381, 19.709355) (-32.645004, 15.951539) knots 0 0 0 0 1 1 1 1
  spline S293 degree 3 poles (-32.645004, 15.951539) (-32.796159, 15.585448) (-32.762994, 15.424728) (-32.599722, 15.337988) knots 0 0 0 0 1 1 1 1
  line L55 (-32.599722, 15.337988) -> (-18.222182, 15.337988)
  spline S294 degree 3 poles (-18.222182, 15.337988) (-17.979186, 15.517842) (-18.090797, 15.749361) (-18.376525, 16.414568) knots 0 0 0 0 1 1 1 1
  spline S295 degree 3 poles (-18.376525, 16.414568) (-20.007333, 20.20555) (-21.361986, 24.089645) (-22.307179, 28.109597) knots 0 0 0 0 1 1 1 1
  spline S296 degree 3 poles (9.47673, 52.701866) (9.979304, 53.606242) (10.020119, 54.566104) (9.730569, 55.52597) knots 0 0 0 0 1 1 1 1
  spline S297 degree 3 poles (9.730569, 55.52597) (9.219704, 57.21737) (7.859953, 58.077102) (5.834353, 58.020978) knots 0 0 0 0 1 1 1 1
  spline S298 degree 3 poles (5.834353, 58.020978) (4.988655, 57.996741) (4.245637, 58.052232) (4.303035, 59.187485) knots 0 0 0 0 1 1 1 1
  spline S299 degree 3 poles (4.303035, 59.187485) (4.331735, 59.760215) (3.928021, 59.975147) (3.487949, 59.976422) knots 0 0 0 0 1 1 1 1
  spline S300 degree 3 poles (3.487949, 59.976422) (1.255709, 59.984076) (-0.976531, 59.940069) (-3.209409, 59.926673) knots 0 0 0 0 1 1 1 1
  spline S301 degree 3 poles (-3.209409, 59.926673) (-3.770021, 59.922848) (-4.341475, 59.757661) (-4.361245, 59.186842) knots 0 0 0 0 1 1 1 1
  spline S302 degree 3 poles (-4.361245, 59.186842) (-4.395048, 58.207206) (-4.793023, 57.92531) (-5.69995, 58.09113) knots 0 0 0 0 1 1 1 1
  spline S303 degree 3 poles (-5.69995, 58.09113) (-5.985038, 58.144066) (-6.298191, 58.056689) (-6.596035, 58.02544) knots 0 0 0 0 1 1 1 1
  spline S304 degree 3 poles (-6.596035, 58.02544) (-9.842987, 57.688054) (-10.802851, 54.657947) (-9.300233, 52.134877) knots 0 0 0 0 1 1 1 1
  spline S305 degree 3 poles (-9.300233, 52.134877) (-7.998518, 49.949832) (-6.489522, 47.888521) (-5.069819, 45.773631) knots 0 0 0 0 1 1 1 1
  spline S306 degree 3 poles (-5.069819, 45.773631) (-4.85361, 45.451553) (-4.791745, 45.109699) (-4.81662, 44.721926) knots 0 0 0 0 1 1 1 1
  spline S307 degree 3 poles (-4.81662, 44.721926) (-4.91739, 43.184234) (-5.010506, 41.647175) (-5.070457, 40.108209) knots 0 0 0 0 1 1 1 1
  spline S308 degree 3 poles (-5.070457, 40.108209) (-5.081298, 39.835874) (-5.117016, 39.627322) (-5.217146, 39.478075) knots 0 0 0 0 1 1 1 1
  line L56 (-5.217146, 39.478075) -> (-6.087081, 39.478075)
  spline S309 degree 3 poles (-6.087081, 39.478075) (-7.14899, 39.478075) (-8.009996, 38.617706) (-8.009996, 37.556435) knots 0 0 0 0 1 1 1 1
  spline S310 degree 3 poles (-8.009996, 37.556435) (-8.009996, 36.592111) (-7.300144, 35.79679) (-6.375359, 35.657752) knots 0 0 0 0 1 1 1 1
  spline S311 degree 3 poles (-6.375359, 35.657752) (-6.34666, 35.650735) (-6.32051, 35.640536) (-6.291809, 35.634152) knots 0 0 0 0 1 1 1 1
  line L57 (-6.291809, 35.634152) -> (-6.087081, 35.634152)
  line L58 (-6.087081, 35.634152) -> (5.85859, 35.634152)
  line L59 (5.85859, 35.634152) -> (6.121358, 35.634152)
  spline S312 degree 3 poles (6.121358, 35.634152) (6.503389, 35.707501) (6.821006, 35.854188) (7.066554, 36.062108) knots 0 0 0 0 1 1 1 1
  spline S313 degree 3 poles (7.066554, 36.062108) (7.074208, 36.067207) (7.081224, 36.073591) (7.088878, 36.079324) knots 0 0 0 0 1 1 1 1
  spline S314 degree 3 poles (7.088878, 36.079324) (7.11439, 36.102281) (7.14054, 36.123973) (7.164134, 36.148205) knots 0 0 0 0 1 1 1 1
  spline S315 degree 3 poles (7.164134, 36.148205) (7.542979, 36.498988) (7.780872, 36.999007) (7.780872, 37.556425) knots 0 0 0 0 1 1 1 1
  spline S316 degree 3 poles (7.780872, 37.556425) (7.780872, 38.617697) (6.919866, 39.478065) (5.858595, 39.478065) knots 0 0 0 0 1 1 1 1
  line L60 (5.858595, 39.478065) -> (5.157035, 39.478065)
  spline S317 degree 3 poles (5.157035, 39.478065) (5.082416, 39.573096) (5.041596, 39.703843) (5.034579, 39.886888) knots 0 0 0 0 1 1 1 1
  spline S318 degree 3 poles (5.034579, 39.886888) (4.96761, 41.665666) (4.90447, 43.444443) (4.818373, 45.221941) knots 0 0 0 0 1 1 1 1
  spline S319 degree 3 poles (4.818373, 45.221941) (4.80179, 45.562515) (4.973994, 45.779363) (5.137902, 46.035752) knots 0 0 0 0 1 1 1 1
  spline S320 degree 3 poles (5.137902, 46.035752) (6.560788, 48.272464) (8.185861, 50.379062) (9.47673, 52.701866) knots 0 0 0 0 1 1 1 1
  spline S321 degree 3 poles (68.902791, 19.494428) (67.698657, 21.970936) (66.672468, 24.505485) (65.910313, 27.166323) knots 0 0 0 0 1 1 1 1
  spline S322 degree 3 poles (65.910313, 27.166323) (65.577388, 28.327725) (65.575481, 29.547168) (65.150075, 30.761501) knots 0 0 0 0 1 1 1 1
  line L61 (65.150075, 30.761501) -> (63.891092, 30.761501)
  spline S323 degree 3 poles (63.891092, 30.761501) (63.393622, 30.744285) (62.89551, 30.747468) (62.39804, 30.761501) knots 0 0 0 0 1 1 1 1
  line L62 (62.39804, 30.761501) -> (60.198324, 30.761501)